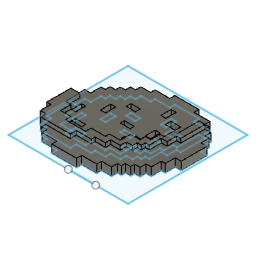
Donut v1 (Autodesk Fusion 360 design; units mm, degrees)
Autodesk Fusion 360 part; units mm, degrees
sketch "donut" plane through (0, 0, 0) normal (0, 0, 1) x (1, 0, 0)
  line L0 (-14.8997, 14.5433) -> (15.1003, 14.5433)
  line L1 (15.1003, 14.5433) -> (15.1003, -15.4567)
  line L2 (15.1003, -15.4567) -> (-14.8997, -15.4567)
  line L3 (-14.8997, -15.4567) -> (-14.8997, 14.5433)
  line L4 (0.1003, -15.4567) -> (7, -15.4567)
  line L5 (-0.5843, 12) -> (5.5, 12)
  line L6 (5.5, 10.7617) -> (9.5, 10.7617)
  line L7 (9.5, 10.7617) -> (9.5, 9.5)
  line L8 (9.5, 9.5) -> (10.5, 9.5)
  line L9 (10.5, 8.5) -> (12, 8.5)
  line L10 (12, 8.5) -> (12, 7)
  line L11 (12, 7) -> (13, 7)
  line L12 (13, 7) -> (13, 5)
  line L13 (13, 5) -> (14.5, 5)
  line L14 (14.5, 5) -> (14.5, -1.5)
  line L15 (13, -1.5) -> (13, -4)
  line L16 (12, -4) -> (12, -6.5)
  line L17 (10.6859, -6.5) -> (10.6859, -8)
  line L18 (9.3046, -8) -> (9.3046, -9)
  line L19 (8, -9) -> (8, -10)
  line L20 (7, -10) -> (7, -11.5)
  line L21 (7, -11.5) -> (4.5, -11.5)
  line L22 (4.5, -11.5) -> (4.5, -12.7202)
  line L23 (4.5, -12.7202) -> (0.6999, -12.7202)
  line L24 (0.6999, -12.7202) -> (0.6999, -14)
  line L25 (0.6999, -14) -> (-5.5, -14)
  line L26 (-5.5, -12.7202) -> (-9.2183, -12.7202)
  line L27 (-9.2183, -11.4974) -> (-10.5, -11.4974)
  line L28 (-10.5, -10.5) -> (-11.7771, -10.5)
  line L29 (-11.7771, -9.1651) -> (-13.2036, -9.1651)
  line L30 (-13.2036, -9.1651) -> (-13.2036, -6.5)
  line L31 (-13.2036, -6.5) -> (-14.2453, -6.5)
  line L32 (-14.2453, -6.5) -> (-14.2453, -0.4567)
  line L33 (-13.2036, -0.4567) -> (-13.2036, 2)
  line L34 (-11.7178, 2) -> (-11.7178, 4.5798)
  line L35 (-10.6328, 4.5798) -> (-10.6328, 5.8155)
  line L36 (-9.2765, 5.8155) -> (-9.2765, 7)
  line L37 (-8, 7) -> (-8, 8.2869)
  line L38 (-6.7448, 8.2869) -> (-6.7448, 9.6131)
  line L39 (-6.7448, 9.6131) -> (-4.3035, 9.6131)
  line L40 (-4.3035, 9.6131) -> (-4.3035, 10.7282)
  line L41 (-4.3035, 10.7282) -> (-0.5843, 10.7282)
  line L42 (-0.5843, 10.7282) -> (-0.5843, 12)
  line L43 (-13.2036, -0.4567) -> (-12, -0.4567)
  line L44 (-12, -0.4567) -> (-12, -4)
  line L45 (-12, -4) -> (-10.6696, -4)
  line L46 (-10.6696, -4) -> (-10.6696, -6.606)
  line L47 (-10.6696, -6.606) -> (-8, -6.606)
  line L48 (-8, -6.606) -> (-8, -8)
  line L49 (-8, -8) -> (-3, -8)
  line L50 (-3, -8) -> (-3, -6.606)
  line L51 (-3, -6.606) -> (0.5755, -6.606)
  line L52 (0.5755, -6.606) -> (0.5755, -5.5901)
  line L53 (0.5755, -5.5901) -> (3.273, -5.5901)
  line L54 (3.273, -5.5901) -> (3.273, -4)
  line L55 (4.4641, -3) -> (5.6551, -3)
  line L56 (5.6551, -3) -> (5.6551, -1.6315)
  line L57 (5.6551, -1.6315) -> (7, -1.6315)
  line L58 (7, -1.6315) -> (7, 0.6805)
  line L59 (7, 0.6805) -> (8, 0.6805)
  line L60 (8, 0.6805) -> (8, 3)
  line L61 (9, 3) -> (9, 8.5)
  line L62 (10.5, 8.5) -> (9, 8.5)
  line L63 (10.5, 8.5) -> (10.5, 2.3621)
  line L64 (10.5, 2.3621) -> (9.4736, 2.3621)
  line L65 (9.4736, 2.3621) -> (9.4736, 0)
  line L66 (9.4736, 0) -> (8, 0)
  line L67 (8, 0) -> (8, -3)
  line L68 (8, -3) -> (7, -3)
  line L69 (7, -3) -> (7, -4)
  line L70 (7, -4) -> (6, -4)
  line L71 (6, -4) -> (6, -5.2048)
  line L72 (4.429, -5.2048) -> (6, -5.2048)
  line L73 (4.429, -6.7111) -> (4.429, -5.2048)
  line L74 (4.429, -6.7111) -> (2, -6.7111)
  line L75 (2, -6.7111) -> (2, -8)
  line L76 (2, -8) -> (-0.5805, -8)
  line L77 (-0.5805, -8) -> (-0.5805, -9)
  line L78 (-0.5805, -9) -> (-4.3289, -9)
  line L79 (-4.3289, -9) -> (-4.3289, -10.5)
  line L80 (-4.3289, -10.5) -> (-10.5, -10.5)
  line L81 (-10.5, -1.5) -> (-9.5, -1.5)
  line L82 (-9.5, -1.5) -> (-9.5, -4)
  line L83 (-9.5, -4) -> (-10.5, -4)
  line L84 (-10.5, -4) -> (-10.5, -1.5)
  line L85 (-6.7666, 2.0722) -> (-5.5, 2.0722)
  line L86 (-5.5, 2.0722) -> (-5.5, -0.5)
  line L87 (-5.5, -0.5) -> (-6.7666, -0.5)
  line L88 (-6.7666, -0.5) -> (-6.7666, 2.0722)
  line L89 (-8, -5.5) -> (-5.5, -5.5)
  line L90 (-5.5, -5.5) -> (-5.5, -6.5)
  line L91 (-5.5, -6.5) -> (-8, -6.5)
  line L92 (-8, -6.5) -> (-8, -5.5)
  line L93 (4.5, 2) -> (5.7276, 2)
  line L94 (5.7276, 2) -> (5.7276, -0.5)
  line L95 (5.7276, -0.5) -> (4.5, -0.5)
  line L96 (4.5, -0.5) -> (4.5, 2)
  line L97 (2, -3) -> (3.273, -3)
  line L98 (3.273, -3) -> (3.273, -4)
  line L99 (3.273, -4) -> (2, -4)
  line L100 (2, -4) -> (2, -3)
  line L101 (3.273, -1.7383) -> (4.4641, -1.7383)
  line L102 (4.4641, -1.7383) -> (4.4641, -3)
  line L103 (4.4641, -3) -> (3.273, -3)
  line L104 (3.273, -3) -> (3.273, -1.7383)
  line L105 (-4.304, 4.7162) -> (-2, 4.7162)
  line L106 (-2, 4.7162) -> (-2, 3.5)
  line L107 (-2, 3.5) -> (-4.304, 3.5)
  line L108 (-4.304, 3.5) -> (-4.304, 4.7162)
  line L109 (2, 8.5) -> (3.2391, 8.5)
  line L110 (3.2391, 8.5) -> (3.2391, 5.9086)
  line L111 (3.2391, 5.9086) -> (2, 5.9086)
  line L112 (2, 5.9086) -> (2, 8.5)
  line L113 (4.5352, 5.9086) -> (7, 5.9086)
  line L114 (7, 5.9086) -> (7, 4.5)
  line L115 (7, 4.5) -> (4.5352, 4.5)
  line L116 (4.5352, 4.5) -> (4.5352, 5.9086)
  line L117 (-1.4423, 0.1714) -> (1.0577, 0.1714)
  line L118 (1.0577, 0.1714) -> (1.0577, -0.8286)
  line L119 (1.0577, -0.8286) -> (-1.4423, -0.8286)
  line L120 (-1.4423, -0.8286) -> (-1.4423, 0.1714)
  line L121 (-11.7771, -10.5) -> (-11.7771, -9.1651)
  line L122 (-13.2036, 2) -> (-11.7178, 2)
  line L123 (-11.7178, 4.5798) -> (-10.6328, 4.5798)
  line L124 (-9.2183, -11.4974) -> (-9.2183, -12.7202)
  line L125 (-5.5, -12.7202) -> (-5.5, -14)
  line L126 (7, -10) -> (8, -10)
  line L127 (8, -9) -> (9.3046, -9)
  line L128 (9.3046, -8) -> (10.6859, -8)
  line L129 (10.6859, -6.5) -> (12, -6.5)
  line L130 (12, -4) -> (13, -4)
  line L131 (13, -1.5) -> (14.5, -1.5)
  line L132 (-10.6328, 5.8155) -> (-9.2765, 5.8155)
  line L133 (-14.2453, -0.4567) -> (-13.2036, -0.4567)
  line L134 (-9.2765, 7) -> (-8, 7)
  line L135 (-8, 8.2869) -> (-6.7448, 8.2869)
  line L136 (5.5, 12) -> (5.5, 10.7617)
  line L137 (10.5, 9.5) -> (10.5, 8.5)
  line L138 (8, 3) -> (9, 3)
  line L139 (-10.5, -11.4974) -> (-10.5, -10.5)
  dimension "d1" = 30
  dimension "d2" = 30
  constraint horizontal L0
  constraint vertical L1
  constraint horizontal L2
  constraint vertical L3
  constraint horizontal L4
  constraint midpoint L2 L4.start
  constraint horizontal L5
  constraint parallel L5 L6
  constraint perpendicular L6 L7
  constraint perpendicular L7 L8
  constraint perpendicular L7 L9
  constraint perpendicular L9 L10
  constraint perpendicular L7 L11
  constraint perpendicular L11 L12
  constraint perpendicular L12 L13
  constraint perpendicular L13 L14
  constraint perpendicular L13 L15
  constraint perpendicular L13 L16
  constraint perpendicular L13 L17
  constraint parallel L17 L18
  constraint parallel L18 L19
  constraint parallel L18 L20
  constraint perpendicular L20 L21
  constraint perpendicular L21 L22
  constraint perpendicular L20 L23
  constraint perpendicular L23 L24
  constraint perpendicular L24 L25
  constraint perpendicular L24 L26
  constraint perpendicular L24 L27
  constraint parallel L27 L28
  constraint parallel L27 L29
  constraint perpendicular L29 L30
  constraint perpendicular L30 L31
  constraint perpendicular L29 L32
  constraint parallel L32 L33
  constraint parallel L33 L34
  constraint parallel L34 L35
  constraint parallel L34 L36
  constraint parallel L34 L37
  constraint parallel L37 L38
  constraint perpendicular L38 L39
  constraint perpendicular L39 L40
  constraint perpendicular L40 L41
  constraint perpendicular L41 L42
  constraint perpendicular L33 L43
  constraint perpendicular L43 L44
  constraint perpendicular L33 L45
  constraint perpendicular L43 L46
  constraint perpendicular L33 L47
  constraint perpendicular L47 L48
  constraint perpendicular L33 L49
  constraint perpendicular L47 L50
  constraint perpendicular L33 L51
  constraint perpendicular L51 L52
  constraint perpendicular L52 L53
  constraint perpendicular L51 L54
  constraint perpendicular L51 L56
  constraint perpendicular L57 L58
  constraint perpendicular L58 L59
  constraint perpendicular L57 L60
  constraint perpendicular L23 L61
  constraint perpendicular L61 L62
  constraint perpendicular L9 L63
  constraint perpendicular L63 L64
  constraint perpendicular L64 L65
  constraint perpendicular L60 L66
  constraint perpendicular L64 L67
  constraint perpendicular L67 L68
  constraint perpendicular L68 L69
  constraint perpendicular L67 L70
  constraint perpendicular L70 L71
  constraint perpendicular L71 L72
  constraint perpendicular L72 L73
  constraint perpendicular L73 L74
  constraint perpendicular L72 L75
  constraint perpendicular L73 L76
  constraint perpendicular L76 L77
  constraint perpendicular L77 L78
  constraint perpendicular L78 L79
  constraint perpendicular L79 L80
  constraint parallel L41 L81
  constraint perpendicular L81 L82
  constraint perpendicular L82 L83
  constraint perpendicular L81 L84
  constraint horizontal L85
  constraint vertical L86
  constraint horizontal L87
  constraint vertical L88
  constraint horizontal L89
  constraint vertical L90
  constraint horizontal L91
  constraint vertical L92
  constraint horizontal L93
  constraint vertical L94
  constraint horizontal L95
  constraint vertical L96
  constraint horizontal L97
  constraint vertical L98
  constraint horizontal L99
  constraint vertical L100
  constraint horizontal L101
  constraint vertical L102
  constraint horizontal L103
  constraint vertical L104
  constraint horizontal L105
  constraint vertical L106
  constraint horizontal L107
  constraint vertical L108
  constraint horizontal L109
  constraint vertical L110
  constraint horizontal L111
  constraint vertical L112
  constraint horizontal L113
  constraint vertical L114
  constraint horizontal L115
  constraint vertical L116
  constraint horizontal L117
  constraint vertical L118
  constraint horizontal L119
  constraint vertical L120
  constraint perpendicular L28 L121
  constraint perpendicular L34 L122
  constraint perpendicular L35 L123
  constraint perpendicular L26 L124
  constraint perpendicular L25 L125
  constraint perpendicular L19 L126
  constraint perpendicular L18 L127
  constraint perpendicular L17 L128
  constraint perpendicular L16 L129
  constraint perpendicular L15 L130
  constraint perpendicular L14 L131
  constraint perpendicular L36 L132
  constraint perpendicular L33 L133
  constraint perpendicular L37 L134
  constraint perpendicular L38 L135
  constraint perpendicular L6 L136
  constraint perpendicular L9 L137
  constraint perpendicular L61 L138
  constraint perpendicular L80 L139
  measures "d1" distance of L0.start L0.end
  measures "d2" distance of L0.start L2.end
extrude "Extrude1" add sketch "donut" along normal blind 2 contours L9 L10 L11 L12 L13 L14 L15 L16 L17 L18 L19 L20 L21 L22 L23 L24 L25 L26 L27 L63 L64 L65 L66 L67 L68 L69 L70 L71 L72 L73 L74 L75 L76 L77 L78 L79 L80 L124 L125 L126 L127 L128 L129 L130 L131 L139 makes body 1
extrude "Extrude2" add sketch "donut" along normal blind 3 contours L28 L29 L30 L31 L32 L43 L44 L45 L46 L47 L48 L49 L50 L51 L52 L53 L54 L55 L56 L57 L58 L59 L60 L61 L62 L63 L64 L65 L66 L67 L68 L69 L70 L71 L72 L73 L74 L75 L76 L77 L78 L79 L80 L98 L103 L121 L133 L138 bodies 1
extrude "Extrude3" add sketch "donut" along normal blind 2 separate body contours L5 L6 L7 L8 L33 L34 L35 L36 L37 L38 L39 L40 L41 L42 L43 L44 L45 L46 L47 L48 L49 L50 L51 L52 L53 L54 L55 L56 L57 L58 L59 L60 L61 L62 L97 L99 L100 L101 L102 L104 L122 L123 L132 L134 L135 L136 L137 L138 makes body 2
